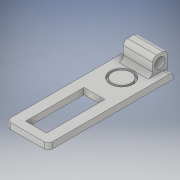
# Autodesk Inventor part: plate1
Saved by Autodesk Inventor 2019 (Build 230136000, 136)
## iProperties
Created: 2021-01-21
Part Number: plate1
Material: Genérico
Document SubType Name: Modeling
Designer: Juan M. Casillas
Density: 1 g/cm^3
Appearance: Valor por defecto
Author: Juan M. Casillas
Autodesk Inventor part; units mm, degrees
ref_plane "YZ Plane" through (0, 0, 0) normal (1, 0, 0) x (0, 1, 0)
ref_plane "XZ Plane" through (0, 0, 0) normal (0, 1, 0) x (-1, 0, 0)
ref_plane "XY Plane" through (0, 0, 0) normal (0, 0, 1) x (1, 0, 0)
sketch "Sketch1" plane through (0, 0, 0) normal (0, 1, 0) x (-1, 0, 0)
  line L0 (10, 30) -> (-10, 30)
  line L1 (-10, 30) -> (-10, -30)
  line L2 (-10, -30) -> (10, -30)
  line L3 (10, -30) -> (10, 30)
  line L4 (10, 30) -> (-10, -30) construction
  line L5 (-10, 30) -> (10, -30) construction
  line L6 (5, 25.9002) -> (-5, 25.9002)
  line L7 (-5, 25.9002) -> (-5, -2.0998)
  line L8 (-5, -2.0998) -> (5, -2.0998)
  line L9 (5, -2.0998) -> (5, 25.9002)
  line L10 (5, 25.9002) -> (-5, -2.0998) construction
  line L11 (-5, 25.9002) -> (5, -2.0998) construction
  circle A0 centre (0, -15.2326) radius 5.5
  point P0 (0, 0)
  point P1 (0, 11.9002)
  dimension "d0" = 20
  dimension "d1" = 60
  dimension "d2" = 10
  dimension "d3" = 28
  dimension "d4" = 11
  constraints: 24 end point, 4 midpoint, 4 parallel, 2 horizontal, 2 perpendicular, 1 centre point
  measures "d0" distance of L2.end L1.end
  measures "d1" distance of L1.end L0.end
  measures "d2" distance of L8.end L7.end
  measures "d3" distance of L7.end L6.end
  measures "d4" diameter of A0
extrude "Extrusion1" add sketch "Sketch1" along normal blind 3
sketch "Sketch2" plane through (0, 3, 0) normal (0, 1, 0) x (1, 0, 0)
  point P0 (0, 0)
sketch "Sketch8" plane through (0, 3, 0) normal (0, 1, 0) x (1, 0, 0)
  line L0 (-10, 30) -> (-10, -30) projected
  line L1 (-10, 30) -> (10, 30)
  line L2 (10, 30) -> (10, 23)
  line L3 (10, 23) -> (-10, 23)
  line L4 (-10, 23) -> (-10, 30)
  point P0 (0, 0)
  dimension "d24" = 20
  dimension "d25" = 7
  constraints: 8 end point, 2 parallel, 1 horizontal, 1 perpendicular
  measures "d24" distance of L2.end L3.end
  measures "d25" distance of L1.end L2.end
extrude "Extrusion7" add sketch "Sketch8" along normal blind 8
sketch "Sketch9" plane through (10, 0, 30) normal (1, 0, 0) x (0, 0, -1)
  line L0 (0, 0) -> (60, 0) projected
  line L1 (60, 0) -> (60, 11) projected
  line L2 (53, 11) -> (60, 11) projected
  line L3 (53, 3) -> (53, 11) projected
  line L4 (0, 3) -> (53, 3) projected
  line L5 (0, 0) -> (0, 3) projected
  circle A0 centre (56.5, 7) radius 2.5
  point P0 (30, 0)
  dimension "d28" = 5
  constraints: 1 centre point
  measures "d28" diameter of A0
extrude "Extrusion8" cut sketch "Sketch9" against normal through all contours A0
sketch "Sketch10" plane through (10, 0, 30) normal (1, 0, 0) x (0, 0, -1)
  circle A0 centre (56.5, 7) radius 2.5 projected
  line L0 (0, 0) -> (60, 0) projected
  line L1 (60, 0) -> (60, 11) projected
  line L2 (53, 11) -> (60, 11) projected
  line L3 (53, 3) -> (53, 11) projected
  line L4 (0, 3) -> (53, 3) projected
  line L5 (0, 0) -> (0, 3) projected
  line L6 (53, 3) -> (53, 11) projected
  line L7 (53, 3) -> (53, 0)
  line L8 (53, 3) -> (0, 3) projected
  line L9 (53, 3) -> (60, 3)
  point P0 (30, 0)
  constraints: 4 end point, 2 perpendicular, 2 point on line
extrude "Extrusion9" cut sketch "Sketch10" against normal blind 3 contours L3 L2 L1 L9
sketch "Sketch12" plane through (-10, 0, -30) normal (-1, 0, 0) x (0, 0, 1)
  circle A0 centre (3.5, 7) radius 2.5 projected
  line L0 (0, 0) -> (60, 0) projected
  line L1 (60, 0) -> (60, 3) projected
  line L2 (7, 3) -> (60, 3) projected
  line L3 (7, 3) -> (7, 11) projected
  line L4 (0, 11) -> (7, 11) projected
  line L5 (0, 0) -> (0, 11) projected
  line L6 (0, 3) -> (7, 3) projected
  line L7 (0, 3) -> (7, 3)
  line L8 (60, 3) -> (0, 3) projected
  point P0 (30, 0)
  constraints: 2 end point, 1 collinear
extrude "Extrusion10" cut sketch "Sketch12" against normal blind 3 contours L5 L4 L3 L6
fillet "Fillet3" radius 2 3 edges at (0, 11, -30) (0, 11, -23) (0, 3, -23)
sketch "Sketch13" plane through (0, 0, 0) normal (0, -1, 0) x (1, 0, 0)
  circle A0 centre (0, -15.2326) radius 5.5 projected
  point P0 (0, 0)
extrude "Extrusion11" add sketch "Sketch13" against normal blind 1.5
sketch "Sketch14" plane through (0, 1.5, -15.2326) normal (0, 1, 0) x (1, 0, 0)
  circle A0 centre (0, 0) radius 5.5 projected
  circle A1 centre (0, 0) radius 4.5
  point P0 (0, -15.2326)
  dimension "d38" = 1
  constraints: 1 centre point
  measures "d38" radial gap between concentric circles of A0 A1
extrude "Extrusion12" add sketch "Sketch14" along normal blind 1.5 contours A1
fillet "Fillet4" radius 2 4 edges at (8.5, 3, -30) (-8.5, 3, -30) (10, 1.5, 30) (-10, 1.5, 30)
sketch "Sketch3" plane through (0, 0, 0) normal (0, -1, 0) x (1, 0, 0)
  circle A0 centre (0, -15.2326) radius 5.5 projected
  point P0 (0, 0)
sketch "Sketch4" plane through (0, 1.5, -15.2326) normal (0, 1, 0) x (1, 0, 0)
  circle A0 centre (0, 0) radius 5.5 projected
  circle A1 centre (0, 0) radius 4.5
  point P0 (0, -15.2326)
  dimension "d9" = 1
  constraints: 1 centre point
  measures "d9" radial gap between concentric circles of A0 A1
sketch "Sketch5" plane through (0, 3, 0) normal (0, 1, 0) x (1, 0, 0)
  line L0 (10, 30) -> (-10, 30) projected
  line L1 (10, -30) -> (10, 30) projected
  line L2 (-10, 30) -> (10, 30)
  line L3 (10, 30) -> (10, 23)
  line L4 (10, 23) -> (-10, 23)
  line L5 (-10, 23) -> (-10, 30)
  point P0 (0, 0)
  dimension "d12" = 7
  constraints: 8 end point, 2 parallel, 1 horizontal, 1 perpendicular, 1 point on line
  measures "d12" distance of L2.end L3.end
sketch "Sketch6" plane through (0, 9, 0) normal (0, 1, 0) x (1, 0, 0)
  line L0 (-10, 30) -> (-10, 23) construction
  line L1 (-10, 23) -> (10, 23) construction
  line L2 (10, 23) -> (10, 30) construction
  line L3 (10, 30) -> (-10, 30) construction
  line L4 (10, 30) -> (-10, 30) projected
  line L5 (-5, 22.9393) -> (5, 22.9393)
  line L6 (5, 22.9393) -> (5, 30)
  line L7 (5, 30) -> (-5, 30)
  line L8 (-5, 30) -> (-5, 22.9393)
  line L9 (-5, 22.9393) -> (5, 30) construction
  line L10 (5, 22.9393) -> (-5, 30) construction
  point P0 (0, 0)
  point P1 (0, 26.4696)
  dimension "d15" = 10
  constraints: 12 end point, 2 midpoint, 2 parallel, 1 horizontal, 1 perpendicular, 1 point on line
  measures "d15" distance of L7.end L6.end
sketch "Sketch7" plane through (-10, 0, -30) normal (-1, 0, 0) x (0, 0, 1)
  arc A0 (2, 9) -> (0, 7) centre (2, 7) ccw construction
  line L0 (0, 0) -> (0, 7) construction
  line L1 (0, 0) -> (60, 0) construction
  line L2 (60, 0) -> (60, 3) construction
  line L3 (7, 3) -> (60, 3) construction
  line L4 (7, 3) -> (7, 7) construction
  line L5 (2, 9) -> (5, 9) construction
  arc A1 (7, 7) -> (5, 9) centre (5, 7) ccw projected
  circle A2 centre (3.5, 5) radius 2.5
  point P0 (30, 0)
  dimension "d20" = 5
  constraints: 1 centre point
  measures "d20" diameter of A2
body "Solid1"
